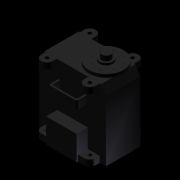
# Autodesk Inventor part: rs405
Saved by Autodesk Inventor 2011 (Build 150239000, 239)
## iProperties
Created: 2009-08-19
Part Number: rs405
Document SubType Name: Modeling
Designer: hajime
Density: 1.60493 g/cm^3
Material: Default
Mass: 66 g
Surface Area: 100.882 cm^2
Volume: 41.1233 cm^3
Author: hajime
Autodesk Inventor part; units mm, degrees
ref_plane "YZ Plane" through (0, 0, 0) normal (1, 0, 0) x (0, 1, 0)
ref_plane "XZ Plane" through (0, 0, 0) normal (0, 1, 0) x (-1, 0, 0)
ref_plane "XY Plane" through (0, 0, 0) normal (0, 0, 1) x (1, 0, 0)
sketch "スケッチ1" plane through (0, 0, 0) normal (0, 0, 1) x (1, 0, 0)
  line L0 (-20.6499, 10.2438) -> (19.8501, 10.2438)
  line L1 (19.8501, 10.2438) -> (19.8501, -10.7562)
  line L2 (19.8501, -10.7562) -> (-20.6499, -10.7562)
  line L3 (-20.6499, -10.7562) -> (-20.6499, 10.2438)
  dimension "d0" = 21
  dimension "d1" = 40.5
  constraints: 8 end point, 2 parallel, 1 horizontal, 1 perpendicular
  measures "d0" distance of L2.end L0.start
  measures "d1" distance of L0.start L0.end
extrude "押し出し1" add sketch "スケッチ1" along normal blind 41.8
sketch "スケッチ2" plane through (0, 0, 41.8) normal (0, 0, 1) x (1, 0, 0)
  line L0 (-20.6499, 10.2438) -> (19.8501, 10.2438) projected
  line L1 (-20.6499, -10.7562) -> (-20.6499, 10.2438) projected
  line L2 (-13.3999, 16.2438) -> (12.6001, 16.2438)
  line L3 (12.6001, 16.2438) -> (12.6001, -16.7562)
  line L4 (12.6001, -16.7562) -> (-13.3999, -16.7562)
  line L5 (-13.3999, -16.7562) -> (-13.3999, 16.2438)
  line L6 (-13.3999, 12.7438) -> (12.6001, 12.7438)
  line L7 (12.6001, 12.7438) -> (12.6001, -13.2562)
  line L8 (12.6001, -13.2562) -> (-13.3999, -13.2562)
  line L9 (-13.3999, -13.2562) -> (-13.3999, 12.7438)
  circle A0 centre (-13.3999, 12.7438) radius 3.5
  circle A1 centre (-13.3999, -13.2562) radius 3.5
  circle A2 centre (12.6001, -13.2562) radius 3.5
  circle A3 centre (12.6001, 12.7438) radius 3.5
  line L10 (-16.8999, 12.7438) -> (-9.8999, 12.7438)
  line L11 (-9.8999, 12.7438) -> (-9.8999, -13.2562)
  line L12 (-9.8999, -13.2562) -> (-16.8999, -13.2562)
  line L13 (-16.8999, -13.2562) -> (-16.8999, 12.7438)
  line L14 (9.1001, 12.7438) -> (16.1001, 12.7438)
  line L15 (16.1001, 12.7438) -> (16.1001, -13.2562)
  line L16 (16.1001, -13.2562) -> (9.1001, -13.2562)
  line L17 (9.1001, -13.2562) -> (9.1001, 12.7438)
  dimension "d4" = 6
  dimension "d5" = 33
  dimension "d6" = 26
  dimension "d7" = 7.25
  dimension "d8" = 26
  dimension "d9" = 2.5
  dimension "d10" = 26
  dimension "d11" = 7
  dimension "d12" = 7
  dimension "d13" = 7
  dimension "d14" = 7
  constraints: 32 end point, 8 parallel, 4 centre point, 4 coincident, 4 collinear, 4 horizontal, 4 perpendicular, 4 tangent, 1 point on line
  measures "d4" distance between parallel lines of L2 L0
  measures "d5" distance of L2.end L3.end
  measures "d6" distance of L2.start L2.end
  measures "d7" distance between parallel lines of L1 L5
  measures "d8" distance of L6.end L7.end
  measures "d9" distance between parallel lines of L0 L6
  measures "d10" distance of L6.start L6.end
  measures "d11" diameter of A0
  measures "d12" diameter of A3
  measures "d13" diameter of A2
  measures "d14" diameter of A1
extrude "押し出し2" add sketch "スケッチ2" against normal blind 3.7 contours L13 A0 L0 | L0 A0 L5 A1 L13 | A0 L10 L5 L0 | L0 L5 A0 | L12 L5 A1 | A1 L5 L12 | A0 L5 L10 | L5 L6 A0 L0 | L0 A0 L5 | A0 L0 L11 A1 L5 | L5 L8 A1 | A1 L8 L5 | A0 L6 L5 | A0 L11 L0 | A2 L8 L3 | L3 L16 A2 | A3 L14 L3 | L3 L6 A3 | L8 A2 L3 | L3 A2 L16 | L17 L0 A3 L3 A2 | A2 L3 A3 L0 L15 | L14 A3 L0 L3 | L3 L0 A3 L6 | L15 L0 A3 | A3 L0 L17 | L3 A3 L0 | L0 A3 L3
sketch "スケッチ3" plane through (0, 0, 41.8) normal (0, 0, 1) x (1, 0, 0)
  line L0 (-20.6499, -10.7562) -> (-20.6499, 10.2438) projected
  line L1 (-9.8999, 10.2438) -> (9.1001, 10.2438) projected
  circle A0 centre (9.5501, -0.2562) radius 4
  dimension "d17" = 10.5
  dimension "d18" = 30.2
  dimension "d19" = 8
  constraints: 1 centre point
  measures "d17" distance from line of L1 A0.centre
  measures "d18" distance from line of A0.centre L0
  measures "d19" diameter of A0
extrude "押し出し3" add sketch "スケッチ3" along normal blind 1.9
sketch "スケッチ4" plane through (9.5501, -0.2562, 43.7) normal (0, 0, 1) x (1, 0, 0)
  circle A0 centre (0, 0) radius 4 projected
  circle A1 centre (0, 0) radius 10.5
  dimension "d22" = 21
  constraints: 1 centre point, 1 coincident
  measures "d22" diameter of A1
extrude "押し出し4" add sketch "スケッチ4" along normal blind 1.9 contours A0 | A1
sketch "スケッチ5" plane through (9.5501, -0.2562, 45.6) normal (0, 0, 1) x (1, 0, 0)
  circle A0 centre (0, 0) radius 10.5 projected
  circle A1 centre (0, 0) radius 4
  dimension "d25" = 8
  constraints: 1 centre point, 1 coincident
  measures "d25" diameter of A1
extrude "押し出し5" add sketch "スケッチ5" along normal blind 1.2 contours A1
sketch "スケッチ6" plane through (9.5501, -0.2562, 46.8) normal (0, 0, 1) x (1, 0, 0)
  circle A0 centre (0, 0) radius 4 projected
  circle A1 centre (0, 0) radius 2.75
  dimension "d28" = 5.5
  constraints: 1 centre point, 1 coincident
  measures "d28" diameter of A1
extrude "押し出し6" add sketch "スケッチ6" along normal blind 3 contours A1
sketch "スケッチ7" plane through (0, 0, 0) normal (0, 0, -1) x (-1, 0, 0)
  line L0 (9.8999, -10.7562) -> (16.8999, -10.7562) projected
  line L1 (9.8999, -13.2562) -> (9.8999, -10.7562) projected
  arc A0 (9.8999, -13.2562) -> (16.8999, -13.2562) centre (13.3999, -13.2562) ccw projected
  line L2 (16.8999, -10.7562) -> (16.8999, -13.2562) projected
  line L3 (16.8999, 10.2438) -> (9.8999, 10.2438) projected
  line L4 (16.8999, 12.7438) -> (16.8999, 10.2438) projected
  arc A1 (16.8999, 12.7438) -> (9.8999, 12.7438) centre (13.3999, 12.7438) ccw projected
  line L5 (9.8999, 10.2438) -> (9.8999, 12.7438) projected
  line L6 (-9.1001, 10.2438) -> (-16.1001, 10.2438) projected
  line L7 (-9.1001, 12.7438) -> (-9.1001, 10.2438) projected
  arc A2 (-9.1001, 12.7438) -> (-16.1001, 12.7438) centre (-12.6001, 12.7438) ccw projected
  line L8 (-16.1001, 10.2438) -> (-16.1001, 12.7438) projected
  line L9 (-16.1001, -10.7562) -> (-9.1001, -10.7562) projected
  line L10 (-16.1001, -13.2562) -> (-16.1001, -10.7562) projected
  arc A3 (-16.1001, -13.2562) -> (-9.1001, -13.2562) centre (-12.6001, -13.2562) ccw projected
  line L11 (-9.1001, -10.7562) -> (-9.1001, -13.2562) projected
  line L12 (13.3999, -16.7562) -> (-12.6001, -16.7562)
  line L13 (-12.6001, -16.7562) -> (-12.6001, 16.2438)
  line L14 (-12.6001, 16.2438) -> (13.3999, 16.2438)
  line L15 (13.3999, 16.2438) -> (13.3999, -16.7562)
  constraints: 8 end point, 2 parallel, 2 point on line, 2 tangent, 1 horizontal, 1 perpendicular
extrude "押し出し7" add sketch "スケッチ7" against normal blind 3.7
sketch "スケッチ8" plane through (0, 0, 0) normal (0, 0, -1) x (-1, 0, 0)
  line L0 (16.8999, -10.7562) -> (20.6499, -10.7562) projected
  line L1 (20.6499, -10.7562) -> (20.6499, 10.2438) projected
  line L2 (9.6499, -17.5562) -> (-8.8501, -17.5562)
  line L3 (-8.8501, -17.5562) -> (-8.8501, 17.0438)
  line L4 (-8.8501, 17.0438) -> (9.6499, 17.0438)
  line L5 (9.6499, 17.0438) -> (9.6499, -17.5562)
  dimension "d33" = 34.6
  dimension "d34" = 6.8
  dimension "d35" = 11
  dimension "d36" = 18.5
  constraints: 8 end point, 2 parallel, 1 horizontal, 1 perpendicular
  measures "d33" distance of L4.end L2.start
  measures "d34" distance between parallel lines of L2 L0
  measures "d35" distance between parallel lines of L5 L1
  measures "d36" distance of L3.end L4.end
extrude "押し出し8" add sketch "スケッチ8" against normal blind 15
sketch "スケッチ9" plane through (19.8501, -10.7562, 0) normal (0, -1, 0) x (1, 0, 0)
  line L0 (-40.5, 0) -> (-40.5, 41.8) projected
  line L1 (-36.75, 0) -> (-40.5, 0) projected
  line L2 (-28.75, 31.6) -> (-11.75, 31.6)
  line L3 (-11.75, 31.6) -> (-11.75, 26.6)
  line L4 (-11.75, 26.6) -> (-28.75, 26.6)
  line L5 (-28.75, 26.6) -> (-28.75, 31.6)
  dimension "d39" = 26.6
  dimension "d40" = 5
  dimension "d41" = 11.75
  dimension "d42" = 17
  constraints: 8 end point, 2 parallel, 1 horizontal, 1 perpendicular
  measures "d39" distance between parallel lines of L1 L4
  measures "d40" distance of L4.end L2.start
  measures "d41" distance between parallel lines of L0 L5
  measures "d42" distance of L2.start L2.end
extrude "押し出し9" add sketch "スケッチ9" along normal blind 6
sketch "スケッチ10" plane through (-20.6499, 10.2438, 41.8) normal (0, 1, 0) x (1, 0, 0)
  line L0 (28.75, 10.2) -> (28.75, 15.2) projected
  line L1 (11.75, 10.2) -> (28.75, 10.2) projected
  line L2 (11.75, 15.2) -> (11.75, 10.2) projected
  line L3 (28.75, 15.2) -> (11.75, 15.2) projected
extrude "押し出し10" add sketch "スケッチ10" along normal blind 6
fillet "フィレット1" radius 1 4 edges at (8.1001, -16.7562, 29.1) (-8.8999, -16.7562, 29.1) (8.1001, 16.2438, 29.1) (-8.8999, 16.2438, 29.1)
sketch "スケッチ11" plane through (-8.8999, -10.7562, 31.6) normal (0, 0, 1) x (1, 0, 0)
  line L0 (1, -6) -> (16, -6) projected
  line L1 (0, 0) -> (17, 0) projected
  line L2 (0, 0) -> (0, -5) projected
  line L3 (1, 0) -> (16, 0)
  line L4 (16, 0) -> (16, -4)
  line L5 (15, -5) -> (2, -5)
  line L6 (1, -4) -> (1, 0)
  line L7 (17, 0) -> (17, -5) projected
  arc A0 (1, -4) -> (2, -5) centre (2, -4) ccw
  arc A1 (15, -5) -> (16, -4) centre (15, -4) ccw
  arc A2 (17, 26) -> (16, 27) centre (16, 26) ccw projected
  line L8 (16, 27) -> (1, 27) projected
  arc A3 (1, 27) -> (0, 26) centre (1, 26) ccw projected
  line L9 (0, 21) -> (0, 26) projected
  line L10 (17, 21) -> (0, 21) projected
  line L11 (17, 21) -> (17, 26) projected
  line L12 (1, 21) -> (16, 21)
  line L13 (16, 21) -> (16, 25)
  line L14 (15, 26) -> (2, 26)
  line L15 (1, 25) -> (1, 21)
  arc A4 (2, 26) -> (1, 25) centre (2, 25) ccw
  arc A5 (16, 25) -> (15, 26) centre (15, 25) ccw
  dimension "d48" = 1
  dimension "d49" = 1
  dimension "d50" = 1
  dimension "d51" = 1
  dimension "d52" = 1
  dimension "d53" = 1
  constraints: 16 end point, 8 point on circle, 8 tangent, 4 centre point, 4 parallel, 2 collinear, 2 equal radius, 2 horizontal, 2 perpendicular, 2 point on line
  measures "d48" distance between parallel lines of L2 L6
  measures "d49" distance between parallel lines of L7 L4
  measures "d50" distance between parallel lines of L0 L5
  measures "d51" radius of A0
  measures "d52" distance between parallel lines of L8 L14
  measures "d53" radius of A4
extrude "押し出し11" cut sketch "スケッチ11" against normal blind 6 contours L1 L4 A1 L5 A0 L6 | L10 L15 A4 L14 A5 L13
sketch "スケッチ12" plane through (0, 0, 41.8) normal (0, 0, 1) x (1, 0, 0)
  arc A0 (-16.8999, -13.2562) -> (-9.8999, -13.2562) centre (-13.3999, -13.2562) ccw projected
  arc A1 (9.1001, -13.2562) -> (16.1001, -13.2562) centre (12.6001, -13.2562) ccw projected
  arc A2 (16.1001, 12.7438) -> (9.1001, 12.7438) centre (12.6001, 12.7438) ccw projected
  arc A3 (-9.8999, 12.7438) -> (-16.8999, 12.7438) centre (-13.3999, 12.7438) ccw projected
  constraints: 4 coincident
hole "穴1" at (-13.3999, 12.7438, 41.8) at (12.6001, 12.7438, 41.8) at (12.6001, -13.2562, 41.8) at (-13.3999, -13.2562, 41.8) direction (0, 0, -1) diameter 2.2 depth 100 tip angle 118
chamfer "面取り1" distance 5 distance2 3 1 edges at (-20.6499, -0.2562, 41.8) measured on face at (-20.6499, -3.7562, 13.9333)
chamfer "面取り2" distance 5 distance2 3 1 edges at (19.8501, -0.2562, 41.8) measured on face at (19.8501, 3.2438, 13.9333)
sketch "スケッチ13" plane through (0, 0, 0) normal (0, 0, -1) x (-1, 0, 0)
  circle A0 centre (-9.5501, -0.2562) radius 4 projected
  constraints: 1 coincident
hole "穴2" at (9.5501, -0.2562, 0) direction (0, 0, 1) diameter 2.459 depth 10 tip angle 118 thread size "M3x0.5" class "6H" standard "ANSI Metric M Profile"
sketch "スケッチ14" plane through (9.5501, -0.2562, 45.6) normal (0, 0, 1) x (1, 0, 0)
  circle A0 centre (0, 0) radius 4 projected
  circle A1 centre (0, 0) radius 2.75 projected
  circle A2 centre (0, 0) radius 7.5
  line L0 (0, 0) -> (7.5, 0)
  line L1 (0, 0) -> (6.9291, 2.8701)
  point P0 (2.8701, 6.9291)
  point P1 (-2.8701, 6.9291)
  point P2 (-6.9291, 2.8701)
  point P3 (-6.9291, -2.8701)
  point P4 (-2.8701, -6.9291)
  point P5 (2.8701, -6.9291)
  point P6 (6.9291, -2.8701)
  dimension "d76" = 15
  dimension "d77" = 22.5
  dimension "d80" = 360
  constraints: 4 end point, 2 coincident, 2 point on circle, 1 centre point, 1 horizontal, 9 other
  measures "d76" diameter of A2
  measures "d77" angle of L1 L0
hole "穴3" at (16.4792, 2.6139, 45.6) at (12.4202, 6.6729, 45.6) at (6.68, 6.6729, 45.6) at (2.621, 2.6139, 45.6) at (2.621, -3.1263, 45.6) at (6.68, -7.1853, 45.6) at (12.4202, -7.1853, 45.6) at (16.4792, -3.1263, 45.6) direction (0, 0, -1) diameter 1.567 depth 2 tip angle 118 thread size "M2x0.4" class "6H" standard "ANSI Metric M Profile"
